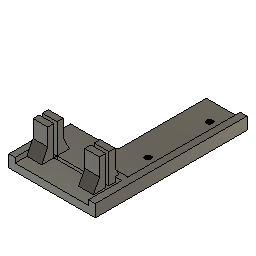
F Machine Base - April 2020 Release v1 (Autodesk Fusion 360 archive; units mm, degrees)
design "Air stroker syringe base mount"
Autodesk Fusion 360 part; units mm, degrees
sketch "Sketch1" plane through (0, 0, 0) normal (0, 0, 1) x (1, 0, 0)
  line L0 (0, 0) -> (0, 73)
  line L1 (0, 73) -> (33, 73)
  line L2 (33, 73) -> (33, -50)
  line L3 (0, 0) -> (-37, 0)
  line L4 (-37, 0) -> (-37, -50)
  line L5 (-37, -50) -> (33, -50)
  circle A0 centre (18, 58) radius 2.5
  circle A1 centre (18, 8) radius 2.5
  line L6 (18, 58) -> (18, 8) construction
  line L7 (-5, -50) -> (-5, 0) construction
  line L8 (-32, -30.5) -> (-20, -30.5)
  line L9 (-20, -30.5) -> (-20, -35.5)
  line L10 (-20, -35.5) -> (-32, -35.5)
  line L11 (-32, -35.5) -> (-32, -30.5)
  line L12 (10, -30.5) -> (22, -30.5)
  line L13 (22, -30.5) -> (22, -35.5)
  line L14 (22, -35.5) -> (10, -35.5)
  line L15 (10, -35.5) -> (10, -30.5)
  line L16 (-32, -23) -> (-20, -23)
  line L17 (-20, -23) -> (-20, -28)
  line L18 (-20, -28) -> (-32, -28)
  line L19 (-32, -28) -> (-32, -23)
  line L20 (10, -23) -> (22, -23)
  line L21 (22, -23) -> (22, -28)
  line L22 (22, -28) -> (10, -28)
  line L23 (10, -28) -> (10, -23)
  line L24 (-20, -28) -> (10, -28)
  line L25 (10, -30.5) -> (10, -28)
  line L26 (10, -30.5) -> (-20, -30.5)
  line L27 (-20, -30.5) -> (-20, -28)
  dimension "d1" = 33
  dimension "d2" = 5
  dimension "d3" = 5
  dimension "d4" = 15
  dimension "d5" = 50
  dimension "d6" = 8
  dimension "d7" = 50
  dimension "d8" = 70
  dimension "d9" = 18
  dimension "d10" = 23
  dimension "d11" = 30
  dimension "d12" = 2.5
  dimension "d13" = 2.5
  dimension "d14" = 12
  dimension "d15" = 12
  dimension "d16" = 36
  dimension "d17" = 5
  dimension "d18" = 5
  constraint coincident L0.start L3.start
  constraint vertical L0
  constraint perpendicular L0 L1
  constraint perpendicular L1 L2
  constraint perpendicular L0 L3
  constraint perpendicular L3 L4
  constraint perpendicular L2 L5
  constraint coincident A0.centre L6.start
  constraint coincident A1.centre L6.end
  constraint vertical L6
  constraint coincident L5 L7.start
  constraint perpendicular L5 L7
  constraint horizontal L8
  constraint vertical L9
  constraint horizontal L10
  constraint vertical L11
  constraint horizontal L12
  constraint vertical L13
  constraint horizontal L14
  constraint vertical L15
  constraint horizontal L16
  constraint vertical L17
  constraint horizontal L18
  constraint vertical L19
  constraint horizontal L20
  constraint vertical L21
  constraint horizontal L22
  constraint vertical L23
  constraint collinear L16 L20
  constraint collinear L18 L22
  constraint collinear L10 L14
  constraint collinear L11 L19
  constraint collinear L9 L17
  constraint collinear L15 L23
  constraint collinear L13 L21
  constraint symmetric L7 L17 L23
  measures "d1" distance of L0.end L1.end
  measures "d2" diameter of A0
  measures "d3" diameter of A1
  measures "d4" distance of L1 A0.centre
  measures "d5" distance of A0.centre A1.centre
  measures "d6" distance of L3 A1.centre
  measures "d7" distance of L3 L5
  measures "d8" distance of L2.end L4.end
  measures "d9" distance of L0 A0.centre
  measures "d10" distance of A1.centre L7
  measures "d11" distance of L9 L15
  measures "d12" distance of L8 L18
  measures "d13" distance of L12 L22
  measures "d14" distance of L16.start L16.end
  measures "d15" distance of L20.start L20.end
  measures "d16" distance of A1.centre L18
  measures "d17" distance of L16.start L18.end
  measures "d18" distance of L8.start L10.end
extrude "Extrude2" add sketch "Sketch1" along normal blind 6 makes body 1
extrude "Extrude1" add sketch "Sketch1" along normal blind 30 separate body contours L16 L17 L18 L19 | L20 L21 L22 L23 | L12 L13 L14 L15 | L8 L9 L10 L11 makes body 2 at (-28, -30.5, 10) makes body 3 at (14, -23, 10) makes body 4 at (-24, -28, 10) makes body 5 at (14, -30.5, 10)
combine "Combine1" operation add target body 1 tool bodies 2 3 4 5
chamfer "Chamfer1" distance 5 distance2 10 4 edges at (16, -35.5, 6) (-26, -35.5, 6) (16, -23, 6) (-26, -23, 6) measured on face at (-19, -7.6667, 6) measured on face at (-19, -7.6667, 6) measured on face at (-19, -7.6667, 6) measured on face at (-19, -7.6667, 6) on bodies 1
sketch "Sketch2" plane through (0, 0, 6) normal (0, 0, 1) x (-1, 0, 0)
  line L0 (20, 18) -> (20, 28)
  line L1 (20, 28) -> (-10, 28)
  line L2 (-10, 28) -> (-10, 18)
  line L3 (-10, 18) -> (-22, 18)
  line L4 (-22, 18) -> (-22, 28)
  line L5 (-22, 28) -> (-10, 28)
  line L6 (-10, 28) -> (-10, 30.5)
  line L7 (-10, 30.5) -> (-22, 30.5)
  line L8 (-22, 30.5) -> (-22, 40.5)
  line L9 (-22, 40.5) -> (-10, 40.5)
  line L10 (-10, 40.5) -> (-10, 30.5)
  line L11 (-10, 30.5) -> (20, 30.5)
  line L12 (20, 30.5) -> (20, 40.5)
  line L13 (20, 40.5) -> (32, 40.5)
  line L14 (32, 40.5) -> (32, 30.5)
  line L15 (32, 30.5) -> (20, 30.5)
  line L16 (20, 30.5) -> (20, 28)
  line L17 (20, 28) -> (32, 28)
  line L18 (32, 28) -> (32, 18)
  line L19 (32, 18) -> (20, 18)
  circle A0 centre (-18, -8) radius 2.5
  circle A1 centre (-18, -58) radius 2.5
  line L20 (0, 0) -> (37, 0)
  line L21 (37, 0) -> (37, 50)
  line L22 (37, 50) -> (-33, 50)
  line L23 (-33, 50) -> (-33, -73)
  line L24 (-33, -73) -> (0, -73)
  line L25 (0, -73) -> (0, 0)
  line L26 (-33, -73) -> (-27.5, -73)
  line L27 (-27.5, -73) -> (-27.5, 50)
  line L28 (-27.5, 50) -> (-33, 50)
  line L29 (-33, 50) -> (-33, -73)
  point P0 (-18, -58)
  dimension "d25" = 9.5
  constraint horizontal L26
  constraint vertical L27
  constraint horizontal L28
  constraint vertical L29
  constraint coincident L22 L27.end
  constraint coincident L23.end L24.start
  measures "d25" horizontal distance of L26.end P0
extrude "Extrude3" add sketch "Sketch2" along normal blind 4 contours L22 L23 L24 L26 L27 L28 L29 bodies 1
sketch "Sketch3" plane through (0, 0, 6) normal (0, 0, 1) x (-1, 0, 0)
  line L0 (-27.5, 50) -> (-27.5, -73)
  line L1 (-27.5, -73) -> (0, -73)
  line L2 (0, -73) -> (0, 0)
  line L3 (0, 0) -> (37, 0)
  line L4 (37, 0) -> (37, 50)
  line L5 (37, 50) -> (-27.5, 50)
  line L6 (20, 18) -> (20, 28)
  line L7 (20, 28) -> (-10, 28)
  line L8 (-10, 28) -> (-10, 18)
  line L9 (-10, 18) -> (-22, 18)
  line L10 (-22, 18) -> (-22, 28)
  line L11 (-22, 28) -> (-10, 28)
  line L12 (-10, 28) -> (-10, 30.5)
  line L13 (-10, 30.5) -> (-22, 30.5)
  line L14 (-22, 30.5) -> (-22, 40.5)
  line L15 (-22, 40.5) -> (-10, 40.5)
  line L16 (-10, 40.5) -> (-10, 30.5)
  line L17 (-10, 30.5) -> (20, 30.5)
  line L18 (20, 30.5) -> (20, 40.5)
  line L19 (20, 40.5) -> (32, 40.5)
  line L20 (32, 40.5) -> (32, 30.5)
  line L21 (32, 30.5) -> (20, 30.5)
  line L22 (20, 30.5) -> (20, 28)
  line L23 (20, 28) -> (32, 28)
  line L24 (32, 28) -> (32, 18)
  line L25 (32, 18) -> (20, 18)
  circle A0 centre (-18, -58) radius 2.5
  circle A1 centre (-18, -8) radius 2.5
  line L26 (-27.5, 18) -> (-10, 18)
  line L27 (-10, 18) -> (-10, 23)
  line L28 (-10, 23) -> (-27.5, 23)
  line L29 (-27.5, 23) -> (-27.5, 18)
  constraint horizontal L26
  constraint vertical L27
  constraint horizontal L28
  constraint vertical L29
  constraint midpoint L8 L27.end
  constraint coincident L0 L26.start
extrude "Extrude5" cut sketch "Sketch3" along normal blind 4 contours L0 L10 L26 L28 L29 | L8 L9 L10 L26 L27 L28 bodies 1
extrude "Extrude4" add sketch "Sketch3" along normal blind 4 contours L0 L10 L26 L28 L29 | L8 L9 L10 L26 L27 L28 bodies 1
extrude "Extrude6" add sketch "Sketch1" along normal blind 2 contours L24 L25 L26 L27 bodies 1
thread "Thread1" "ISO Metric profile 5.0 M5x0.8 6H" major diameter 5.12 minor diameter 4.234 pitch 0.8 angle 60 modelled right hand crest width 0.2219 on face at (20.4969, 7.8754, 4) crest through (20.117, 8, 0.2) on face at (15.6508, 57.1449, 4) crest through (20.117, 58, 0.2) on bodies 1
sketch "Sketch4" plane through (0, 0, 6) normal (0, 0, 1) x (-1, 0, 0)
  line L0 (-27.5, 23) -> (-22, 23)
  line L1 (-22, 23) -> (-22, 28)
  line L2 (-22, 28) -> (-10, 28)
  line L3 (-10, 28) -> (-10, 30.5)
  line L4 (-10, 30.5) -> (-22, 30.5)
  line L5 (-22, 30.5) -> (-22, 40.5)
  line L6 (-22, 40.5) -> (-10, 40.5)
  line L7 (-10, 40.5) -> (-10, 30.5)
  line L8 (-10, 30.5) -> (20, 30.5)
  line L9 (20, 30.5) -> (20, 40.5)
  line L10 (20, 40.5) -> (32, 40.5)
  line L11 (32, 40.5) -> (32, 30.5)
  line L12 (32, 30.5) -> (20, 30.5)
  line L13 (20, 30.5) -> (20, 28)
  line L14 (20, 28) -> (32, 28)
  line L15 (32, 28) -> (32, 18)
  line L16 (32, 18) -> (20, 18)
  line L17 (20, 18) -> (20, 28)
  line L18 (20, 28) -> (-10, 28)
  line L19 (-10, 28) -> (-10, 18)
  line L20 (-10, 18) -> (-27.5, 18)
  line L21 (-27.5, 18) -> (-27.5, -73)
  line L22 (-27.5, -73) -> (0, -73)
  line L23 (0, -73) -> (0, 0)
  line L24 (0, 0) -> (37, 0)
  line L25 (37, 0) -> (37, 50)
  line L26 (37, 50) -> (-27.5, 50)
  line L27 (-27.5, 50) -> (-27.5, 23)
  spline S0 degree 3 poles (-19.6199, -59.3629) (-19.8211, -59.1688) (-19.9816, -58.9366) (-20.2111, -58.4143) (-20.274, -58.1276) (-20.2886, -57.5351) (-20.2361, -57.2349) (-20.0168, -56.6603) (-19.8483, -56.393) (-19.5013, -56.0234) (-19.3523, -55.8984) (-19.0252, -55.6831) (-18.8477, -55.5943) (-18.6617, -55.527) knots 0 0 0 0 0.083865 0.083865 0.170995 0.170995 0.261388 0.261388 0.355043 0.355043 0.412991 0.412991 0.47212 0.47212 0.47212 0.47212
  arc A0 (-17.3383, -55.527) -> (-18.6617, -55.527) centre (-18, -58) ccw
  spline S1 degree 3 poles (-17.3383, -55.527) (-17.031, -55.6383) (-16.748, -55.8075) (-16.2724, -56.2391) (-16.0816, -56.4941) (-15.8151, -57.0538) (-15.7382, -57.3513) (-15.7055, -57.9481) (-15.7458, -58.2413) (-15.8981, -58.6794) (-15.9727, -58.8335) (-16.1544, -59.1176) (-16.2601, -59.2472) (-16.3801, -59.3629) knots 0 0 0 0 0.098035 0.098035 0.192799 0.192799 0.284291 0.284291 0.372508 0.372508 0.423853 0.423853 0.474023 0.474023 0.474023 0.474023
  arc A1 (-19.6199, -59.3629) -> (-16.3801, -59.3629) centre (-18, -58) ccw
  spline S2 degree 3 poles (-19.6199, -9.3629) (-19.8211, -9.1688) (-19.9816, -8.9366) (-20.2111, -8.4143) (-20.274, -8.1276) (-20.2886, -7.5351) (-20.2361, -7.2349) (-20.0168, -6.6603) (-19.8483, -6.393) (-19.5013, -6.0234) (-19.3523, -5.8984) (-19.0252, -5.6831) (-18.8477, -5.5943) (-18.6617, -5.527) knots 0 0 0 0 0.083865 0.083865 0.170995 0.170995 0.261388 0.261388 0.355043 0.355043 0.412991 0.412991 0.47212 0.47212 0.47212 0.47212
  arc A2 (-17.3383, -5.527) -> (-18.6617, -5.527) centre (-18, -8) ccw
  spline S3 degree 3 poles (-17.3383, -5.527) (-17.031, -5.6383) (-16.748, -5.8075) (-16.2724, -6.2391) (-16.0816, -6.4941) (-15.8151, -7.0538) (-15.7382, -7.3513) (-15.7055, -7.9481) (-15.7458, -8.2413) (-15.8981, -8.6794) (-15.9727, -8.8335) (-16.1544, -9.1176) (-16.2601, -9.2472) (-16.3801, -9.3629) knots 0 0 0 0 0.098035 0.098035 0.192799 0.192799 0.284291 0.284291 0.372508 0.372508 0.423853 0.423853 0.474023 0.474023 0.474023 0.474023
  arc A3 (-19.6199, -9.3629) -> (-16.3801, -9.3629) centre (-18, -8) ccw
  line L28 (37, 50) -> (32, 50)
  line L29 (32, 50) -> (32, 12)
  line L30 (32, 12) -> (37, 12)
  line L31 (37, 12) -> (37, 50)
  constraint horizontal L28
  constraint vertical L29
  constraint horizontal L30
  constraint vertical L31
  constraint coincident L25.end L26.start
extrude "Extrude7" add sketch "Sketch4" along normal blind 4 contours L11 L15 L25 L26 L28 L29 L30 L31 bodies 1
chamfer "Chamfer2" distance 3 angle 45 1 edges at (0, 0, 3) on bodies 1
